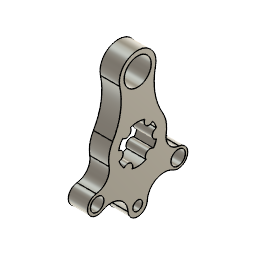
1.1 (Autodesk Fusion 360 design; units mm, degrees)
part number: 2025-10-07-10-13-13-699
Autodesk Fusion 360 part; units mm, degrees
sketch "Sketch1" plane through (0, 0, 0) normal (1, 0, 0) x (0, 1, 0)
  line L0 (0, 77.8292) -> (0, -65)
  line L1 (0, 77.8292) -> (0, -35)
  circle A0 centre (0, 65) radius 14
  circle A1 centre (-41.8386, -32.9309) radius 7
  circle A2 centre (0, -55) radius 5
  arc A3 (-25.8286, 15.2605) -> (-18.5525, 60.9006) centre (-80.0686, 47.3077) ccw
  arc A4 (18.5525, 60.9006) -> (25.8286, 15.2605) centre (80.0686, 47.3077) ccw
  arc A5 (-42.8128, -22.9785) -> (-29.5161, -5.3666) centre (-44.2741, -8.0498) ccw
  arc A6 (-42.8128, -22.9785) -> (-36.612, -41.4564) centre (-41.8386, -32.9309) ccw
  arc A7 (-9.9875, -55.5003) -> (-36.612, -41.4564) centre (-27.4656, -56.3759) ccw
  arc A8 (29.5161, -5.3666) -> (42.8128, -22.9785) centre (44.2741, -8.0498) ccw
  arc A9 (36.612, -41.4564) -> (42.8128, -22.9785) centre (41.8386, -32.9309) ccw
  arc A10 (36.612, -41.4564) -> (9.9875, -55.5003) centre (27.4656, -56.3759) ccw
  circle A11 centre (41.8386, -32.9309) radius 7.5
  arc A12 (-9.9875, -55.5003) -> (9.9875, -55.5003) centre (0, -55) ccw
  arc A13 (-25.8286, 15.2605) -> (-29.5161, -5.3666) centre (0, 0) ccw
  arc A14 (29.5161, -5.3666) -> (25.8286, 15.2605) centre (0, 0) ccw
  arc A15 (18.5525, 60.9006) -> (-18.5525, 60.9006) centre (0, 65) ccw
  arc A16 (-15.3974, 12.764) -> (-7.3687, 18.5931) centre (-11.7502, 16.1843) ccw
  arc A17 (7.3687, 18.5931) -> (15.3974, 12.764) centre (11.7502, 16.1843) ccw
  arc A18 (7.3687, 18.5931) -> (-7.3687, 18.5931) centre (0, 0) ccw
  arc A19 (19.375, 4.9608) -> (19.375, -4.9608) centre (20, 0) ccw
  arc A20 (19.375, 4.9608) -> (15.3974, 12.764) centre (0, 0) ccw
  arc A21 (16.2483, -11.6616) -> (8.6447, -18.0352) centre (12.848, -15.3274) ccw
  arc A22 (16.2483, -11.6616) -> (19.375, -4.9608) centre (0, 0) ccw
  arc A23 (-5.4599, -19.2403) -> (-14.0345, -14.2489) centre (-10.0617, -17.2848) ccw
  arc A24 (-5.4599, -19.2403) -> (8.6447, -18.0352) centre (0, 0) ccw
  arc A25 (-19.1065, -5.9111) -> (-19.5963, 3.9983) centre (-19.9756, -0.9872) ccw
  arc A26 (-15.3974, 12.764) -> (-19.5963, 3.9983) centre (0, 0) ccw
  arc A27 (-19.1065, -5.9111) -> (-14.0345, -14.2489) centre (0, 0) ccw
  dimension "d1" = 28
  dimension "d2" = 38
  dimension "d3" = 60
  dimension "d4" = 40
  dimension "d5" = 14
  dimension "d6" = 20
  dimension "d7" = 10
  dimension "d8" = 126
  dimension "d9" = 126
  dimension "d10" = 30
  dimension "d11" = 35
  dimension "d12" = 15
  dimension "d13" = 10
  dimension "d14" = 10
  dimension "d15" = 10
  dimension "d16" = 10
  dimension "d17" = 10
  dimension "d18" = 10
  constraint vertical L0
  constraint coincident L0 L1.end
  constraint coincident L1 A0.centre
  constraint concentric A0 A15
  constraint coincident A13.centre A14.centre
  constraint concentric A1 A6
  constraint coincident L0 A2.centre
  constraint concentric A2 A12
  constraint tangent A3 A15
  constraint tangent A3 A13
  constraint tangent A4 A15
  constraint tangent A4 A13
  constraint tangent A5 A13
  constraint tangent A5 A6
  constraint tangent A6 A7
  constraint tangent A7 A12
  constraint symmetric L0 A5.end A8.start
  constraint symmetric L0 A5.start A8.end
  constraint symmetric L0 A5 A8
  constraint symmetric L0 A6.end A9.start
  constraint symmetric L0 A6 A9
  constraint symmetric L0 A7.start A10.end
  constraint symmetric L0 A7 A10
  constraint concentric A9 A11
  constraint concentric A13 A14
  constraint coincident A16.centre A26
  constraint coincident A25.centre A26
  constraint coincident A23.centre A26
  constraint coincident A17.centre A26
  constraint coincident A19.centre A26
  constraint coincident A21.centre A26
  constraint coincident A17.start A26
  constraint concentric A18 A26
  constraint coincident A19.start A26
  constraint concentric A20 A26
  constraint coincident A21.start A26
  constraint concentric A22 A26
  constraint coincident A23.start A26
  constraint concentric A24 A26
  constraint coincident A25.start A26
  constraint concentric A26 A27
  measures "d1" diameter of A0
  measures "d2" diameter of A15
  measures "d3" diameter of A13
  measures "d4" diameter of A26
  measures "d5" diameter of A1
  measures "d6" diameter of A6
  measures "d7" diameter of A2
  measures "d8" diameter of A3
  measures "d9" diameter of A4
  measures "d10" diameter of A5
  measures "d11" diameter of A7
  measures "d12" diameter of A11
  measures "d13" diameter of A16
  measures "d14" diameter of A25
  measures "d15" diameter of A23
  measures "d16" diameter of A17
  measures "d17" diameter of A19
  measures "d18" diameter of A21
extrude "Extrude1" add sketch "Sketch1" along normal blind 20
